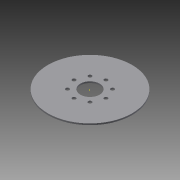
# Autodesk Inventor part: S25-60L Aluminum Sprocket (am-0237)
Saved by Autodesk Inventor 2015 (Build 190159000, 159)
## iProperties
Created: 2015-01-18
Part Number: S25-60L Aluminum Sprocket (am-0237)
Material: Generic
Document SubType Name: Modeling
Designer: chapale16
Density: 1 g/cm^3
Appearance: Default
Author: chapale16
Autodesk Inventor part; units mm, degrees
ref_plane "YZ Plane" through (0, 0, 0) normal (1, 0, 0) x (0, 1, 0)
ref_plane "XZ Plane" through (0, 0, 0) normal (0, 1, 0) x (-1, 0, 0)
ref_plane "XY Plane" through (0, 0, 0) normal (0, 0, 1) x (1, 0, 0)
sketch "Sketch1" plane through (0, 0, 0) normal (0, 1, 0) x (-1, 0, 0)
  circle A0 centre (0, 0) radius 62.3951
  circle A1 centre (0, 0) radius 14.2812
  dimension "d0" = 124.7902
  dimension "d1" = 28.5623
  constraints: 2 centre point, 2 coincident
  measures "d0" diameter of A0
  measures "d1" diameter of A1
extrude "Extrusion1" add sketch "Sketch1" along normal blind 2.2098
sketch "Sketch2" plane through (0, 2.2098, 0) normal (0, 1, 0) x (1, 0, 0)
  circle A0 centre (0, 0) radius 14.2812 projected
  circle A1 centre (-23.6791, 0) radius 2.667
  circle A2 centre (-16.7437, 16.7437) radius 2.667
  circle A3 centre (0, 23.6791) radius 2.667
  circle A4 centre (16.7437, 16.7437) radius 2.667
  circle A5 centre (23.6791, 0) radius 2.667
  circle A6 centre (16.7437, -16.7437) radius 2.667
  circle A7 centre (0, -23.6791) radius 2.667
  circle A8 centre (-16.7437, -16.7437) radius 2.667
  dimension "d8" = 360
  constraints: 8 centre point, 2 coincident, 22 other
extrude "Extrusion2" cut sketch "Sketch2" against normal through all contours A1 | A2 | A3 | A4 | A5 | A6 | A7 | A8
body "Solid1"
